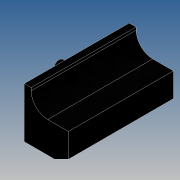
# Autodesk Inventor part: Boton de extraccion
Saved by Autodesk Inventor 2016 (Build 200138000, 138)
## iProperties
Created: 2016-05-25
Part Number: Boton de extraccion
Material: ABS Plastic
Document SubType Name: Modeling
Designer: Familia
Density: 1.06 g/cm^3
Appearance: Black
Mass: 5.91279 g
Surface Area: 38.6354 cm^2
Volume: 5.5781 cm^3
Author: Familia
Autodesk Inventor part; units mm, degrees
ref_plane "YZ Plane" through (0, 0, 0) normal (1, 0, 0) x (0, 1, 0)
ref_plane "XZ Plane" through (0, 0, 0) normal (0, 1, 0) x (-1, 0, 0)
ref_plane "XY Plane" through (0, 0, 0) normal (0, 0, 1) x (1, 0, 0)
sketch "Sketch2" plane through (0, 0, 0) normal (0, 1, 0) x (-1, 0, 0)
  line L0 (0, 18.2) -> (0, 0)
  line L1 (0, 0) -> (-11, 0)
  line L2 (-11, 0) -> (-16, 2.5)
  line L3 (-16, 2.5) -> (-16, 11.2)
  line L4 (-16, 11.2) -> (-2.5, 11.2)
  line L5 (-2.5, 11.2) -> (-2.5, 18.2)
  line L6 (-2.5, 18.2) -> (0, 18.2)
  dimension "d0" = 18.2
  dimension "d1" = 11.2
  dimension "d2" = 2.5
  dimension "d3" = 16
  dimension "d4" = 5
  dimension "d5" = 2.5
  constraints: 14 end point, 4 perpendicular, 1 parallel, 1 vertical
  measures "d0" distance of L0.start L0.end
  measures "d1" distance between parallel lines of L1 L4
  measures "d2" distance of L5.end L0.start
  measures "d3" distance between parallel lines of L3 L0
  measures "d4" horizontal distance of L1.end L2.end
  measures "d5" vertical distance of L1.end L2.end
extrude "Extrusion1" add sketch "Sketch2" along normal mid plane 38
fillet "Fillet1" radius 6 1 edges at (2.5, 0, 11.2)
sketch "Sketch3" plane through (0, -19, 18.2) normal (-1, 0, 0) x (0, 0, 1)
  line L0 (-9.7, 35.9) -> (-16.2, 35.9)
  line L1 (-16.2, 35.9) -> (-16.2, 2.1)
  line L2 (-16.2, 2.1) -> (-9.7, 2.1)
  line L3 (-9.7, 2.1) -> (-9.7, 35.9)
  line L4 (-18.2, 19) -> (-16.2, 19) construction
  line L5 (-18.2, 38) -> (-18.2, 0) construction
  line L6 (0, 0) -> (-18.2, 0) construction
  line L7 (-18.2, 38) -> (0, 38) construction
  dimension "d9" = 2
  dimension "d10" = 33.8
  dimension "d11" = 6.5
  constraints: 10 end point, 2 horizontal, 2 parallel, 1 midpoint, 1 perpendicular
  measures "d9" distance between parallel lines of L5 L1
  measures "d10" distance of L2.end L0.start
  measures "d11" distance of L0.start L0.end
extrude "Extrusion2" cut sketch "Sketch3" against normal blind 10
sketch "Sketch4" plane through (0, -19, 18.2) normal (-1, 0, 0) x (0, 0, 1)
  circle A0 centre (-7.2, 19) radius 2
  line L0 (-7.2, 19) -> (-18.2, 19) construction
  dimension "d14" = 4
  dimension "d15" = 11
  constraints: 2 end point, 1 centre point, 1 horizontal
  measures "d14" diameter of A0
  measures "d15" distance of L0.end L0.start
extrude "Extrusion3" add sketch "Sketch4" along normal blind 6.4
sketch "Sketch5" plane through (0, -19, 18.2) normal (-1, 0, 0) x (0, 0, 1)
  line L0 (-9.7, 21.5) -> (-11.7, 21.5)
  line L1 (-11.7, 16.5) -> (-9.7, 16.5)
  line L2 (-9.7, 16.5) -> (-9.7, 21.5)
  line L3 (-16.2, 35.9) -> (-9.7, 35.9) construction
  line L4 (-9.7, 2.1) -> (-16.2, 2.1) construction
  line L5 (-9.7, 35.9) -> (-9.7, 2.1) construction
  line L6 (-12.95, 35.9) -> (-12.95, 2.1) construction
  line L7 (-18.2, 19) -> (-9.9, 19)
  line L8 (-11.7, 18.5) -> (-9.9, 18.5)
  line L9 (-9.9, 18.5) -> (-9.9, 19.5)
  line L10 (-9.9, 19.5) -> (-11.7, 19.5)
  line L11 (-11.7, 21.5) -> (-11.7, 19.5)
  line L12 (-11.7, 18.5) -> (-11.7, 16.5)
  line L13 (-16.2, 21.5) -> (-14.2, 21.5)
  line L14 (-14.2, 16.5) -> (-16.2, 16.5)
  line L15 (-16.2, 16.5) -> (-16.2, 21.5)
  line L16 (-14.2, 18.5) -> (-16, 18.5)
  line L17 (-16, 18.5) -> (-16, 19.5)
  line L18 (-16, 19.5) -> (-14.2, 19.5)
  line L19 (-14.2, 21.5) -> (-14.2, 19.5)
  line L20 (-14.2, 18.5) -> (-14.2, 16.5)
  point P0 (-16, 19)
  dimension "d19" = 5
  dimension "d20" = 2
  dimension "d21" = 2.5
  dimension "d22" = 1
  dimension "d23" = 1.8
  constraints: 36 end point, 9 symmetric about line, 5 perpendicular, 3 horizontal, 3 midpoint, 3 parallel, 1 collinear, 1 point on line
  measures "d19" distance of L1.end L0.start
  measures "d20" distance of L1.start L1.end
  measures "d21" distance between parallel lines of L7 L0
  measures "d22" distance between parallel lines of L10 L8
  measures "d23" distance of L8.start L8.end
extrude "Extrusion4" add sketch "Sketch5" against normal up to next
body "Solid1"
